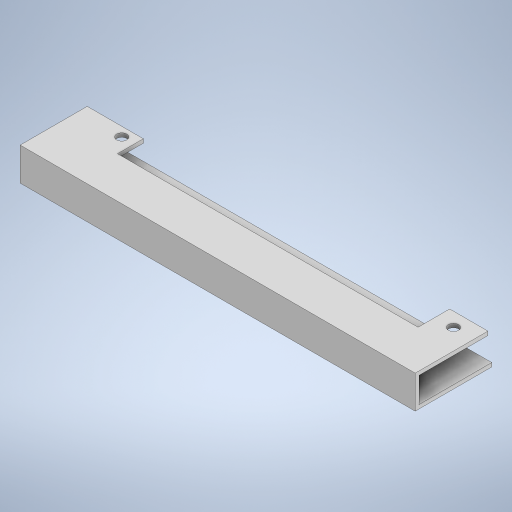
# Autodesk Inventor part: CO-1-01-jetsonMount
Saved by Autodesk Inventor 2023 (Build 270158000, 158)
## iProperties
Created: 2023-01-24
Part Number: CO-1-01-jetsonMount
Material: Generic
Document SubType Name: Modeling
Designer: t205b
Density: 1 g/cm^3
Appearance: Default
Author: t205b
Autodesk Inventor part; units mm, degrees
ref_plane "YZ Plane" through (0, 0, 0) normal (1, 0, 0) x (0, 1, 0)
ref_plane "XZ Plane" through (0, 0, 0) normal (0, 1, 0) x (-1, 0, 0)
ref_plane "XY Plane" through (0, 0, 0) normal (0, 0, 1) x (1, 0, 0)
sketch "Sketch1" plane through (0, 0, 0) normal (0, 1, 0) x (-1, 0, 0)
  line L0 (13.8415, 5.1768) -> (-89.2585, 5.1768)
  line L1 (-89.2585, 5.1768) -> (-89.2585, -12.8232)
  line L2 (-89.2585, -12.8232) -> (-79.2585, -12.8232)
  line L3 (-79.2585, -12.8232) -> (-79.2585, -4.5732)
  line L4 (-79.2585, -4.5732) -> (-0.8085, -4.5732)
  line L5 (-0.8085, -4.5732) -> (-0.8085, -11.3232)
  line L6 (-0.8085, -11.3232) -> (13.8415, -11.3232)
  line L7 (13.8415, -11.3232) -> (13.8415, 5.1768)
  circle A0 centre (2.4165, -8.8982) radius 1.325
  circle A1 centre (-83.9335, -9.1482) radius 1.325
  line L8 (13.8415, 5.1768) -> (-89.2585, 5.1768)
  line L9 (-89.2585, 5.1768) -> (-89.2585, 6.1768)
  line L10 (-89.2585, 6.1768) -> (13.8415, 6.1768)
  line L11 (13.8415, 6.1768) -> (13.8415, 5.1768)
  point P0 (0, 0)
  dimension "d0" = 2.65
  dimension "d1" = 2.65
  dimension "d2" = 103.1
  dimension "d3" = 14.65
  dimension "d4" = 10
  dimension "d5" = 18
  dimension "d6" = 16.5
  dimension "d7" = 14.075
  dimension "d8" = 11.425
  dimension "d9" = 9.75
  dimension "d10" = 14.325
  dimension "d11" = 5.325
  dimension "d14" = 1
  constraints: 24 end point, 8 perpendicular, 2 centre point, 2 horizontal, 2 parallel, 1 other
  measures "d0" diameter of A0
  measures "d1" diameter of A1
  measures "d2" distance between parallel lines of L7 L1
  measures "d3" distance between parallel lines of L7 L5
  measures "d4" distance between parallel lines of L3 L1
  measures "d5" distance between parallel lines of L0 L2
  measures "d6" distance between parallel lines of L0 L6
  measures "d7" distance from line of L0 A0.centre
  measures "d8" distance from line of L7 A0.centre
  measures "d9" distance between parallel lines of L0 L4
  measures "d10" distance from line of L0 A1.centre
  measures "d11" distance from line of L1 A1.centre
  measures "d14" distance of L8.end L9.end
extrude "Extrusion1" add sketch "Sketch1" along normal blind 1
extrude "Extrusion2" add sketch "Sketch1" against normal blind 7.6 contours L0 L9 L10 L11
sketch "Sketch3" plane through (89.2585, 0, 5.1768) normal (0, 0, -1) x (-1, 0, 0)
  line L0 (103.1, -7.6) -> (0, -7.6) projected
  line L1 (103.1, -7.6) -> (103.1, 1) projected
  line L2 (0, -7.6) -> (103.1, -7.6)
  line L3 (103.1, -7.6) -> (103.1, -6.6)
  line L4 (103.1, -6.6) -> (0, -6.6)
  line L5 (0, -6.6) -> (0, -7.6)
  point P0 (89.2585, 0)
  dimension "d17" = 1
  constraints: 8 end point, 2 parallel, 1 horizontal, 1 perpendicular, 1 point on line
  measures "d17" distance between parallel lines of L0 L4
extrude "Extrusion3" add sketch "Sketch3" along normal blind 19
body "Solid1"
